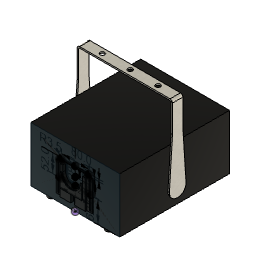
KVANT Clubmax 6000 w Safetyscan (Autodesk Fusion 360 design; units mm, degrees)
part number: Open
Autodesk Fusion 360 part; units mm, degrees
sketch "Body base" plane through (0, 0, 0) normal (0, 0, 1) x (1, 0, 0) in component "Case Body"
  line L0 (-127.7, -158.05) -> (127.7, -158.05)
  line L1 (127.7, -158.05) -> (127.7, 158.05)
  line L2 (127.7, 158.05) -> (-127.7, 158.05)
  line L3 (-127.7, 158.05) -> (-127.7, -158.05)
  line L4 (-127.7, -158.05) -> (127.7, 158.05) construction
  line L5 (127.7, -158.05) -> (-127.7, 158.05) construction
  dimension "d1" = 316.1
  dimension "d2" = 255.4
  constraint horizontal L0
  constraint perpendicular L0 L1
  constraint parallel L0 L2
  constraint parallel L1 L3
  constraint coincident L4 origin
  constraint coincident L5 origin
  measures "d1" distance of L0.end L1.end
  measures "d2" distance of L1.end L2.end
extrude "Extrude1" add sketch "Body base" along normal blind 157.8 makes body 1 in component "Case Body"
sketch "Aperature" plane through (0, -158.05, 0) normal (0, -1, 0) x (1, 0, 0) in component "Case Body"
  line L0 (-127.7, 0) -> (127.7, 0)
  line L1 (127.7, 0) -> (127.7, 157.8)
  line L2 (127.7, 157.8) -> (-127.7, 157.8)
  line L3 (-127.7, 157.8) -> (-127.7, 0)
  line L4 (0, 157.8) -> (0, 0) construction
  line L5 (-36.5, 114) -> (36.5, 114)
  line L6 (40, 110.5) -> (40, 65.5)
  line L7 (36.5, 62) -> (-36.5, 62)
  line L8 (-40, 65.5) -> (-40, 110.5)
  arc A0 (-36.5, 114) -> (-40, 110.5) centre (-36.5, 110.5) ccw
  arc A1 (40, 110.5) -> (36.5, 114) centre (36.5, 110.5) ccw
  arc A2 (36.5, 62) -> (40, 65.5) centre (36.5, 65.5) ccw
  arc A3 (-40, 65.5) -> (-36.5, 62) centre (-36.5, 65.5) ccw
  line L9 (-40, 109) -> (40, 109)
  line L10 (-46, 64) -> (46, 64) construction
  point P0 (-40, 114)
  point P1 (40, 114)
  point P2 (-40, 62)
  point P3 (0, 114)
  point P4 (0, 114)
  point P5 (46, 108)
  point P6 (46, 64)
  point P7 (-46, 64)
  point P8 (-46, 108)
  point P9 (0, 64)
  point P10 (0, 86)
  dimension "d5" = 80
  dimension "d6" = 52
  dimension "d7" = 62
  dimension "d8" = 3.5
  dimension "d9" = 5
  dimension "d18" = 92
  dimension "d19" = 44
  dimension "d20" = 6
  dimension "d81" = 28
  constraint midpoint L2 L4.start
  constraint coincident L4.end origin
  constraint horizontal L5
  constraint vertical L6
  constraint horizontal L7
  constraint vertical L8
  constraint coincident L4 P4
  constraint coincident L5 P4
  constraint coincident P0 L5
  constraint coincident P0 L8
  constraint tangent L5 A0
  constraint tangent L8 A0
  constraint coincident P1 L5
  constraint coincident P1 L6
  constraint tangent L5 A1
  constraint tangent L6 A1
  constraint equal A0 A1
  constraint tangent L6 A2
  constraint tangent L7 A2
  constraint equal A0 A2
  constraint coincident P2 L7
  constraint coincident P2 L8
  constraint tangent L7 A3
  constraint tangent L8 A3
  constraint equal A0 A3
  constraint midpoint L5 P4
  constraint coincident L8 L9.start
  constraint coincident L6 L9.end
  constraint perpendicular L6 L9
  constraint coincident P7 L10.start
  constraint coincident P6 L10.end
  constraint horizontal L10
  constraint horizontal P5 P8
  constraint vertical P5 P6
  constraint vertical P7 P8
  constraint midpoint L10 P9
  constraint coincident L4 P9
  constraint coincident L4 P10
  measures "d5" distance of P0 P1
  measures "d6" distance of P0 P2
  measures "d7" distance of L0 L7
  measures "d8" radius of A0
  measures "d9" distance of L5 L9
  measures "d18" distance of P7 P6
  measures "d19" distance of P5 P6
  measures "d20" distance of L5 P5
  measures "d81" distance of P4 P10
extrude "Extrude2" cut sketch "Aperature" against normal blind 1.5 contours L5 L6 L8 A0 A1 L9 bodies 1 in component "Case Body"
extrude "Extrude3" cut sketch "Aperature" against normal blind 4 contours L6 L7 L8 A2 A3 L9 bodies 1 in component "Case Body"
sketch "Glass" plane through (0, -154.05, 0) normal (0, -1, 0) x (1, 0, 0) in component "Case Body"
  arc A0 (-40, 65.5) -> (-36.5, 62) centre (-36.5, 65.5) ccw
  line L0 (-36.5, 62) -> (36.5, 62)
  arc A1 (36.5, 62) -> (40, 65.5) centre (36.5, 65.5) ccw
  line L1 (40, 65.5) -> (40, 109)
  line L2 (40, 109) -> (-40, 109)
  line L3 (-40, 109) -> (-40, 65.5)
  line L4 (-29.5, 109) -> (29.5, 109)
  line L5 (29.5, 109) -> (29.5, 64)
  line L6 (29.5, 64) -> (-29.5, 64)
  line L7 (-29.5, 64) -> (-29.5, 109)
  line L8 (40, 109) -> (-40, 109)
  point P0 (0, 109)
  point P1 (0, 109)
  dimension "d14" = 59
  dimension "d15" = 45
  constraint horizontal L4
  constraint vertical L5
  constraint horizontal L6
  constraint vertical L7
  constraint midpoint L4 P1
  constraint midpoint L8 P1
  constraint coincident P1 P0
  measures "d14" distance of L4.start L4.end
  measures "d15" distance of L4.start L6.end
extrude "Extrude4" cut sketch "Glass" against normal blind 3.5 contours L2 L4 L5 L6 L7 L8 bodies 1 in component "Case Body"
hole "Hole1" at (46, -158.05, 108) at (46, -158.05, 64) at (-46, -158.05, 108) at (-46, -158.05, 64) direction (0, 1, 0) diameter 3.4 depth 10 tip angle 180 bodies 1 in component "Case Body"
sketch "Aperature knob positions" plane through (0, -158.05, 0) normal (0, -1, 0) x (1, 0, 0) in component "Case Body"
  circle A0 centre (-46, 108) radius 1.7
  circle A1 centre (46, 108) radius 1.7
  circle A2 centre (46, 64) radius 1.7
  circle A3 centre (-46, 64) radius 1.7
  line L0 (-127.7, 0) -> (127.7, 0)
  line L1 (127.7, 0) -> (127.7, 157.8)
  line L2 (127.7, 157.8) -> (-127.7, 157.8)
  line L3 (-127.7, 157.8) -> (-127.7, 0)
  line L4 (40, 110.5) -> (40, 65.5)
  arc A4 (36.5, 62) -> (40, 65.5) centre (36.5, 65.5) ccw
  line L5 (36.5, 62) -> (-36.5, 62)
  arc A5 (-40, 65.5) -> (-36.5, 62) centre (-36.5, 65.5) ccw
  line L6 (-40, 65.5) -> (-40, 110.5)
  arc A6 (-36.5, 114) -> (-40, 110.5) centre (-36.5, 110.5) ccw
  line L7 (-36.5, 114) -> (36.5, 114)
  arc A7 (40, 110.5) -> (36.5, 114) centre (36.5, 110.5) ccw
  line L8 (0, 6) -> (0, 54) construction
  circle A8 centre (0, 54) radius 5
  circle A9 centre (0, 6) radius 5
  dimension "d24" = 48
  dimension "d25" = 6
  dimension "d26" = 10
  dimension "d27" = 10
  constraint vertical L8
  constraint vertical origin L8.start
  constraint coincident L8.end A8.centre
  constraint coincident L8.start A9.centre
  measures "d24" distance of L8.start L8.end
  measures "d25" distance of origin L8.start
  measures "d26" diameter of A8
  measures "d27" diameter of A9
extrude "Extrude5" add sketch "Aperature knob positions" along normal blind 6 separate body contours A8 | A9 makes body 2 at (4.9752, -160.05, 53.5022) makes body 3 at (4.9752, -160.05, 5.5022) in component "Case Body"
sketch "Profile" plane through (0, 0, 0) normal (1, 0, 0) x (0, 1, 0) in component "Yoke"
  circle A0 centre (-0.55, 48.4) radius 24
  line L0 (158.05, 0) -> (158.05, 157.8)
  line L1 (-158.05, 0) -> (158.05, 0)
  line L2 (-15.55, 274.6) -> (14.45, 274.6)
  line L3 (14.45, 274.6) -> (14.45, 189.6)
  line L4 (14.45, 189.6) -> (23.4009, 49.935)
  line L5 (-24.5009, 49.935) -> (-15.55, 189.6)
  line L6 (-15.55, 189.6) -> (-15.55, 274.6)
  point P0 (-0.55, 274.6)
  dimension "d30" = 48
  dimension "d31" = 158.6
  dimension "d32" = 48.4
  dimension "d33" = 30
  dimension "d34" = 226.2
  dimension "d35" = 85
  constraint horizontal L2
  constraint perpendicular L2 L3
  constraint coincident A0 L4.end
  constraint coincident A0 L5.start
  constraint vertical L6
  constraint midpoint L2 P0
  constraint vertical A0.centre P0
  constraint horizontal L3.end L5.end
  constraint tangent A0 L4
  constraint tangent A0 L5
  measures "d30" diameter of A0
  measures "d31" distance of A0.centre L0
  measures "d32" distance of A0.centre L1
  measures "d33" distance of L2.start L2.end
  measures "d34" distance of A0.centre L2
  measures "d35" distance of L2.end L3.end
extrude "Extrude1'" add sketch "Profile" along normal blind 4 from surface at 133.2 separate body makes body 4 in component "Yoke"
extrude "Extrude2'" add sketch "Profile" against normal blind 4 from surface at -133.2 separate body makes body 5 in component "Yoke"
sketch "Top holes" plane through (0, 0, 274.6) normal (0, 0, 1) x (-1, 0, 0) in component "Yoke"
  line L0 (-133.2, -14.45) -> (-133.2, 15.55) construction
  line L1 (-133.2, 15.55) -> (-137.2, 15.55)
  line L2 (-137.2, 15.55) -> (-137.2, -14.45)
  line L3 (-137.2, -14.45) -> (-133.2, -14.45)
  line L4 (133.2, 15.55) -> (133.2, -14.45)
  line L5 (133.2, -14.45) -> (-137.2, -14.45)
  line L6 (-137.2, -14.45) -> (-137.2, 15.55)
  line L7 (-137.2, 15.55) -> (133.2, 15.55)
  line L8 (133.2, 15.55) -> (133.2, -14.45)
  circle A0 centre (80, 0) radius 6.65
  circle A1 centre (0, 0) radius 6.65
  circle A2 centre (-80, 0) radius 6.65
  dimension "d44" = 13.3
  dimension "d47" = 80
  dimension "d48" = 0
  constraint horizontal L5
  constraint vertical L6
  constraint horizontal L7
  constraint vertical L8
  constraint coincident L1.end L2.start
  constraint coincident L4.end L5.start
  constraint coincident A1.centre origin
  measures "d44" diameter of A0
extrude "Extrude3'" add sketch "Top holes" against normal blind 4 bodies 4 5 in component "Yoke"
fillet "Fillet1" radius 3 1 edges at (133.2, -0.55, 270.6) on bodies 4 in component "Yoke"
fillet "Fillet1" radius 7 1 edges at (137.2, -0.55, 274.6) on bodies 4 in component "Yoke"
fillet "Fillet1" radius 7 1 edges at (-137.2, -0.55, 274.6) on bodies 4 in component "Yoke"
fillet "Fillet1" radius 3 1 edges at (-133.2, -0.55, 270.6) on bodies 4 in component "Yoke"
sketch "Feet" plane through (0, 0, 0) normal (0, 0, -1) x (1, 0, 0) in component "Case Body"
  line L0 (-127.7, 158.05) -> (-127.7, -158.05)
  line L1 (-127.7, -158.05) -> (127.7, -158.05)
  line L2 (127.7, -158.05) -> (127.7, 158.05)
  line L3 (127.7, 158.05) -> (-127.7, 158.05)
  circle A0 centre (-82.7, 143.55) radius 12.5
  line L4 (0, -2.5) -> (0, -20)
  circle A1 centre (82.7, 143.55) radius 12.5
  line L5 (20, 0) -> (2.5, 0)
  circle A2 centre (82.7, -143.55) radius 12.5
  circle A3 centre (-82.7, -143.55) radius 12.5
  dimension "d53" = 25
  dimension "d54" = 45
  dimension "d55" = 2
  constraint symmetric A0 L4 A1
  constraint symmetric A0 L5 A3
  constraint symmetric A1 L5 A2
  measures "d53" diameter of A0
  measures "d54" distance of L0 A0.centre
  measures "d55" distance of L3 A0
extrude "Extrude6" add sketch "Feet" along normal blind 10.2 draft -15 contours A0 | A1 | A2 | A3 bodies 1 in component "Case Body"
sketch "Base" plane through (0, -158.05, 0) normal (0, -1, 0) x (1, 0, 0) in component "SafetyScan Bracket"
  circle A0 centre (-46, 108) radius 1.7
  circle A1 centre (46, 108) radius 1.7
  circle A2 centre (46, 64) radius 1.7
  circle A3 centre (-46, 64) radius 1.7
  line L0 (-127.7, 0) -> (127.7, 0)
  line L1 (127.7, 0) -> (127.7, 157.8)
  line L2 (127.7, 157.8) -> (-127.7, 157.8)
  line L3 (-127.7, 157.8) -> (-127.7, 0)
  line L4 (40, 110.5) -> (40, 65.5)
  arc A4 (36.5, 62) -> (40, 65.5) centre (36.5, 65.5) ccw
  line L5 (36.5, 62) -> (-36.5, 62) construction
  arc A5 (-40, 65.5) -> (-36.5, 62) centre (-36.5, 65.5) ccw
  line L6 (-40, 65.5) -> (-40, 110.5)
  arc A6 (-36.5, 114) -> (-40, 110.5) centre (-36.5, 110.5) ccw
  line L7 (-36.5, 114) -> (36.5, 114)
  arc A7 (40, 110.5) -> (36.5, 114) centre (36.5, 110.5) ccw
  line L8 (-51.85, 105.55) -> (51.85, 105.55)
  line L9 (51.85, 105.55) -> (51.85, 22.05)
  line L10 (51.85, 22.05) -> (-51.85, 22.05)
  line L11 (-51.85, 22.05) -> (-51.85, 105.55)
  line L12 (44.35, 101.15) -> (44.35, 26.45)
  arc A8 (44.35, 26.45) -> (47.65, 26.45) centre (46, 26.45) ccw
  line L13 (47.65, 26.45) -> (47.65, 101.15)
  arc A9 (47.65, 101.15) -> (44.35, 101.15) centre (46, 101.15) ccw
  line L14 (46, 102.8) -> (46, 24.8) construction
  line L15 (-28.45, 105.55) -> (-28.45, 88)
  arc A10 (-28.45, 88) -> (28.45, 88) centre (0, 88) ccw
  line L16 (28.45, 88) -> (28.45, 105.55)
  line L17 (-5.4, 22.05) -> (-5.4, 46.15)
  arc A11 (5.4, 46.15) -> (-5.4, 46.15) centre (0, 46.15) ccw
  line L18 (5.4, 46.15) -> (5.4, 22.05)
  line L19 (40, 109) -> (-40, 109)
  line L20 (0, 88) -> (0, 46.15) construction
  line L21 (-44.35, 101.15) -> (-44.35, 26.45)
  arc A12 (-47.65, 26.45) -> (-44.35, 26.45) centre (-46, 26.45) ccw
  line L22 (-47.65, 26.45) -> (-47.65, 101.15)
  arc A13 (-44.35, 101.15) -> (-47.65, 101.15) centre (-46, 101.15) ccw
  point P0 (47.65, 63.8)
  point P1 (51.85, 63.8)
  point P2 (0, 105.55)
  dimension "d58" = 103.7
  dimension "d59" = 83.5
  dimension "d60" = 78
  dimension "d61" = 3.3
  dimension "d62" = 4.2
  dimension "d63" = 56.9
  dimension "d64" = 46
  dimension "d65" = 10.8
  dimension "d66" = 29.5
  dimension "d67" = 21
  constraint horizontal L8
  constraint vertical L9
  constraint horizontal L10
  constraint vertical L11
  constraint tangent L12 A8
  constraint tangent A8 L13
  constraint parallel L12 L13
  constraint tangent L13 A9
  constraint tangent L12 A9
  constraint midpoint A9 L14.start
  constraint midpoint A8 L14.end
  constraint parallel L4 L14
  constraint midpoint L13 P0
  constraint midpoint L9 P1
  constraint horizontal P0 P1
  constraint midpoint L8 P2
  constraint vertical P2 origin
  constraint coincident L8 L15.start
  constraint perpendicular L8 L15
  constraint tangent L15 A10
  constraint coincident L8 L16.end
  constraint tangent A10 L16
  constraint perpendicular L8 L16
  constraint vertical origin A10.centre
  constraint coincident L10 L17.start
  constraint perpendicular L10 L17
  constraint tangent L17 A11
  constraint coincident L10 L18.end
  constraint tangent A11 L18
  constraint perpendicular L10 L18
  constraint vertical origin A11.centre
  constraint coincident A10.centre L20.start
  constraint coincident A11.centre L20.end
  constraint symmetric L12.start L20 L21.start
  constraint symmetric L12.end L20 L21.end
  constraint symmetric A8.end L20 A12.start
  constraint symmetric L13.end L20 L22.end
  constraint symmetric A8 L20 A12
  constraint symmetric A9 L20 A13
  measures "d58" distance of L8.start L8.end
  measures "d59" distance of L8.start L10.end
  measures "d60" distance of L14.start L14.end
  measures "d61" distance of L12 L13
  measures "d62" distance of L9 L13
  measures "d63" distance of L15 L16
  measures "d65" distance of L17 L18
  measures "d67" distance of A10.centre L19
extrude "Extrude1''" add sketch "Base" along normal blind 3.2 separate body contours L8 L9 L10 L11 L15 A10 L16 L17 A11 L18 makes body 6 in component "SafetyScan Bracket"
sketch "Raised" plane through (0, -161.25, 0) normal (0, -1, 0) x (1, 0, 0) in component "SafetyScan Bracket"
  arc A0 (-44.35, 63.5907) -> (-44.35, 64.4093) centre (-46, 64) ccw
  line L0 (-44.35, 63.5907) -> (-44.35, 26.45)
  arc A1 (-47.65, 26.45) -> (-44.35, 26.45) centre (-46, 26.45) ccw
  line L1 (-47.65, 26.45) -> (-47.65, 63.5907)
  arc A2 (-47.65, 64.4093) -> (-47.65, 63.5907) centre (-46, 64) ccw
  line L2 (-47.65, 64.4093) -> (-47.65, 101.15)
  arc A3 (-44.35, 101.15) -> (-47.65, 101.15) centre (-46, 101.15) ccw
  line L3 (-44.35, 101.15) -> (-44.35, 64.4093)
  arc A4 (47.65, 101.15) -> (44.35, 101.15) centre (46, 101.15) ccw
  line L4 (47.65, 101.15) -> (47.65, 64.4093)
  arc A5 (47.65, 63.5907) -> (47.65, 64.4093) centre (46, 64) ccw
  line L5 (47.65, 63.5907) -> (47.65, 26.45)
  arc A6 (44.35, 26.45) -> (47.65, 26.45) centre (46, 26.45) ccw
  line L6 (44.35, 26.45) -> (44.35, 63.5907)
  arc A7 (44.35, 64.4093) -> (44.35, 63.5907) centre (46, 64) ccw
  line L7 (44.35, 64.4093) -> (44.35, 101.15)
  line L8 (-5.4, 22.05) -> (-5.4, 46.15)
  arc A8 (5.4, 46.15) -> (-5.4, 46.15) centre (0, 46.15) ccw
  line L9 (5.4, 46.15) -> (5.4, 22.05)
  line L10 (5.4, 22.05) -> (51.85, 22.05)
  line L11 (51.85, 22.05) -> (51.85, 105.55)
  line L12 (51.85, 105.55) -> (28.45, 105.55)
  line L13 (28.45, 105.55) -> (28.45, 88)
  arc A9 (-28.45, 88) -> (28.45, 88) centre (0, 88) ccw
  line L14 (-28.45, 88) -> (-28.45, 105.55)
  line L15 (-28.45, 105.55) -> (-51.85, 105.55)
  line L16 (-51.85, 105.55) -> (-51.85, 22.05)
  line L17 (-51.85, 22.05) -> (-5.4, 22.05)
  line L18 (-36.4, 105.55) -> (-36.4, 22.05)
  line L19 (36.4, 105.55) -> (36.4, 22.05)
  line L20 (-36.4, 105.55) -> (36.4, 105.55) construction
  point P0 (0, 105.55)
  dimension "d70" = 72.8
  constraint coincident L15 L18.start
  constraint coincident L17 L18.end
  constraint perpendicular L17 L18
  constraint coincident L12 L19.start
  constraint coincident L10 L19.end
  constraint perpendicular L10 L19
  constraint midpoint L20 P0
  constraint vertical P0 origin
  measures "d70" distance of L18 L19
extrude "Extrude2''" add sketch "Raised" along normal blind 4.4 contours L8 A8 L9 L10 L12 L13 A9 L14 L15 L17 L18 L19 bodies 6 in component "SafetyScan Bracket"
sketch "Lens holder" plane through (0, -165.65, 0) normal (0, -1, 0) x (1, 0, 0) in component "SafetyScan Bracket"
  line L0 (28.45, 105.55) -> (28.45, 88)
  arc A0 (-28.45, 88) -> (28.45, 88) centre (0, 88) ccw construction
  line L1 (-28.45, 88) -> (-28.45, 105.55)
  line L2 (-28.45, 105.55) -> (-36.4, 105.55)
  line L3 (-36.4, 105.55) -> (-36.4, 22.05)
  line L4 (-36.4, 22.05) -> (-5.4, 22.05)
  line L5 (-5.4, 22.05) -> (-5.4, 46.15)
  arc A1 (5.4, 46.15) -> (-5.4, 46.15) centre (0, 46.15) ccw
  line L6 (5.4, 46.15) -> (5.4, 22.05)
  line L7 (5.4, 22.05) -> (36.4, 22.05)
  line L8 (36.4, 22.05) -> (36.4, 105.55)
  line L9 (36.4, 105.55) -> (28.45, 105.55)
  line L10 (-31.25, 48.8) -> (31.25, 48.8)
  line L11 (31.25, 48.8) -> (31.25, 90)
  line L12 (31.25, 90) -> (-31.25, 90)
  line L13 (-31.25, 90) -> (-31.25, 48.8)
  arc A2 (-27.1, 88) -> (27.1, 88) centre (0, 88) ccw
  line L14 (27.1, 88) -> (27.1, 90)
  line L15 (-27.1, 88) -> (-27.1, 90)
  point P0 (0, 90)
  dimension "d73" = 62.5
  dimension "d74" = 41.2
  dimension "d76" = 12.1
  dimension "d77" = 54.2
  constraint horizontal L10
  constraint vertical L11
  constraint horizontal L12
  constraint vertical L13
  constraint midpoint L12 P0
  constraint vertical A0.centre P0
  constraint horizontal A2.start A2.end
  constraint coincident L12 L14.end
  constraint perpendicular L12 L14
  constraint coincident L12 L15.end
  constraint tangent A2 L15
  constraint coincident A0.centre A2.centre
  constraint vertical L15
  measures "d73" distance of L10.start L10.end
  measures "d74" distance of L10.start L12.end
  measures "d76" distance of L10 A2
  measures "d77" distance of A2.start A2.end
extrude "Extrude3''" add sketch "Lens holder" along normal blind 2.2 from surface at 3 separate body contours A1 L10 L11 L12 L13 A2 L14 L15 | A1 L10 makes body 7 in component "SafetyScan Bracket"
component "Case Body" placed x (1, 0, 0) y (0, 1, 0) z (0, 0, 1) at (0, 0, 0)
component "Yoke" placed x (1, 0, 0) y (0, 1, 0) z (0, 0, 1) at (0, 0, 0)
component "SafetyScan Bracket" placed x (1, 0, 0) y (0, 1, 0) z (0, 0, 1) at (0, 0, 0)
hidden bodies 2
equation "d27 = d26"
equation "d36 = ( ( ( 274.4 / 2 ) * 1 mm ) - 4 mm )"
equation "d39 = -( ( ( 274.4 / 2 ) * 1 mm ) - 4 mm )"
equation "d75 = ( 51 / 2 ) * 1 mm"
named bodies: "Body", "Aperature knob up", "Aperature knob down"
